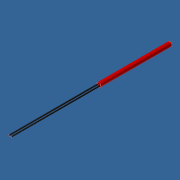
# Autodesk Inventor part: 3618K448
Saved by Autodesk Inventor 2012 SP1 (Build 160190100, 190)
## iProperties
Created: 2012-04-04
Part Number: 3618K448
Material: Default
Vendor: MCMASTER
Document SubType Name: Modeling
Designer: NEGRASHOVI
Density: 1 g/cm^3
Mass: 12.5023 g
Surface Area: 76.7854 cm^2
Volume: 12.5023 cm^3
Description: Cartridge Heater High Temp, 3/8" Dia, 6", 120 VAC, 400W
RuleStatus: InUse
AfterDocSave0: file://Part Number Cleaner
SURFACE ROUGHNESS: N/A
SPECIAL FINISH: NONE
ALTERED ITEM PART NUMBER: N/A
ALTERED ITEM VENDOR: N/A
ALTERED ITEM DESCRIPTION: N/A
Author: NEGRASHOVI
Revision Number: 0
Autodesk Inventor part; units mm, degrees
ref_plane "YZ Plane" through (0, 0, 0) normal (1, 0, 0) x (0, 1, 0)
ref_plane "XZ Plane" through (0, 0, 0) normal (0, 1, 0) x (-1, 0, 0)
ref_plane "XY Plane" through (0, 0, 0) normal (0, 0, 1) x (1, 0, 0)
sketch "Sketch1" plane through (0, 0, 0) normal (0, 0, 1) x (1, 0, 0)
  circle A0 centre (0, 0) radius 4.699
  dimension "d0" = 9.398
  constraints: 1 centre point, 1 coincident
  measures "d0" diameter of A0
extrude "Extrusion1" add sketch "Sketch1" along normal blind 152.4
sketch "Sketch2" plane through (0, 0, 152.4) normal (0, 0, 1) x (1, 0, 0)
  circle A0 centre (0, 0) radius 4.699 construction
  line L0 (-4.699, 0) -> (4.699, 0)
  circle A1 centre (2.54, 0) radius 1.27
  circle A2 centre (-2.54, 0) radius 1.27
  dimension "d3" = 2.54
  dimension "d4" = 2.54
  dimension "d5" = 2.54
  dimension "d6" = 2.54
  constraints: 2 centre point, 2 end point, 2 point on circle, 2 point on line, 1 horizontal, 1 midpoint
  measures "d3" diameter of A1
  measures "d4" diameter of A2
  measures "d5" distance of A2.centre point (0, 0)
  measures "d6" distance of A1.centre point (0, 0)
extrude "Extrusion2" add sketch "Sketch2" along normal blind 190.5
equation "\"d3\" = d4"
equation "\"d6\" = d5"
body "Solid1"
